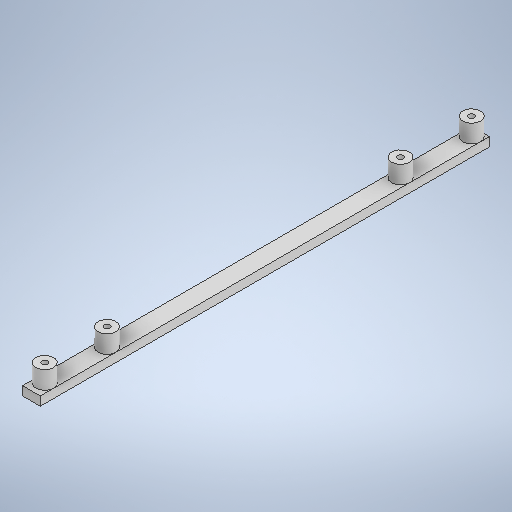
# Autodesk Inventor part: HS MOGO Ramp Jig
Saved by Autodesk Inventor 2025.2 (Build 292293000, 293)
## iProperties
Created: 2025-04-04
Part Number: HS MOGO Ramp Jig
Material: Generic
Document SubType Name: Modeling
Designer: avere
Density: 1 g/cm^3
Appearance: Default
Author: avere
Autodesk Inventor part; units mm, degrees
ref_plane "YZ Plane" through (0, 0, 0) normal (1, 0, 0) x (0, 1, 0)
ref_plane "XZ Plane" through (0, 0, 0) normal (0, 1, 0) x (-1, 0, 0)
ref_plane "XY Plane" through (0, 0, 0) normal (0, 0, 1) x (1, 0, 0)
sketch "Sketch1" plane through (0, 0, 0) normal (0, 1, 0) x (-1, 0, 0)
  line L0 (6.35, 0) -> (-6.35, 0)
  line L1 (-6.35, 0) -> (-6.35, -317.5)
  line L2 (-6.35, -317.5) -> (6.35, -317.5)
  line L3 (6.35, -317.5) -> (6.35, 0)
  circle A0 centre (0, -6.35) radius 2.0955
  circle A1 centre (0, -311.15) radius 2.0955
  circle A2 centre (0, -50.8) radius 2.0955
  circle A3 centre (0, -260.35) radius 2.0955
  point P0 (0, 0)
  dimension "d0" = 12.7
  dimension "d1" = 317.5
  dimension "d2" = 4.191
  constraints: 8 end point, 4 centre point, 2 parallel, 1 horizontal, 1 perpendicular
  measures "d0" distance of L2.end L1.end
  measures "d1" distance of L1.end L0.end
  measures "d2" diameter of A0
extrude "Extrusion1" add sketch "Sketch1" against normal blind 6.35
sketch "Sketch2" plane through (0, -6.35, 0) normal (0, -1, 0) x (1, 0, 0)
  line L0 (6.35, 0) -> (-6.35, 0) projected
  line L1 (-3.175, 0) -> (3.175, 0)
  line L2 (3.175, 0) -> (3.175, -317.5)
  line L3 (3.175, -317.5) -> (-3.175, -317.5)
  line L4 (-3.175, -317.5) -> (-3.175, 0)
  point P0 (0, 0)
  constraints: 8 end point, 2 parallel, 1 horizontal, 1 perpendicular, 1 point on line
extrude "Extrusion2" cut sketch "Sketch2" against normal blind 3.175
sketch "Sketch3" plane through (0, 0, 0) normal (0, 1, 0) x (1, 0, 0)
  circle A0 centre (0, 6.35) radius 6.35
  circle A1 centre (0, 50.8) radius 6.35
  line L0 (-6.35, 317.5) -> (-6.35, 0) projected
  circle A2 centre (0, 260.35) radius 6.35
  circle A3 centre (0, 311.15) radius 6.35
  circle A4 centre (0, 50.8) radius 2.0955 projected
  circle A5 centre (0, 6.35) radius 2.0955 projected
  circle A6 centre (0, 260.35) radius 2.0955 projected
  circle A7 centre (0, 311.15) radius 2.0955 projected
  point P0 (0, 0)
  constraints: 4 centre point, 1 tangent
extrude "Extrusion3" add sketch "Sketch3" along normal blind 12.7
sketch "Sketch4" plane through (6.35, -6.35, 0) normal (0, 0, 1) x (1, 0, 0)
  line L0 (0, 6.35) -> (0, 0) projected
  line L1 (0, 0) -> (-12.7, 0)
  line L2 (-12.7, 0) -> (-12.7, 6.35)
  line L3 (-12.7, 6.35) -> (0, 6.35)
  line L4 (0, 6.35) -> (0, 0)
  point P0 (-6.35, 6.35)
  constraints: 8 end point, 2 parallel, 1 horizontal, 1 perpendicular
extrude "Extrusion4" add sketch "Sketch4" along normal blind 3.175
body "Solid1"
